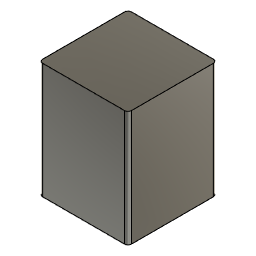
Body v1 (Autodesk Fusion 360 design; units mm, degrees)
Autodesk Fusion 360 part; units mm, degrees
sketch "Sketch1" plane through (0, 0, 0) normal (0, 0, 1) x (1, 0, 0)
  line L0 (25, -25) -> (-25, -25)
  line L1 (-25, -25) -> (-25, 25)
  line L2 (-25, 25) -> (25, 25)
  line L3 (25, 25) -> (25, -25)
  line L4 (25, -25) -> (-25, 25) construction
  line L5 (-25, -25) -> (25, 25) construction
  dimension "d1" = 50
  dimension "d2" = 50
  constraint horizontal L0
  constraint perpendicular L0 L1
  constraint parallel L0 L2
  constraint parallel L1 L3
  constraint coincident L4 origin
  constraint coincident L5 origin
  measures "d1" distance of L1.end L2.end
  measures "d2" distance of L0.end L1.end
extrude "Extrude1" add sketch "Sketch1" along normal blind 65
fillet "Fillet1" radius 2 4 edges at (-25, -25, 32.5) (25, -25, 32.5) (-25, 25, 32.5) (25, 25, 32.5)
shell "Shell1" thickness 1.6 removed faces 1 at (7.6667, -8.3333, 65)
sketch "Sketch2" plane through (0, 0, 65) normal (0, 0, 1) x (-1, 0, 0)
  arc A0 (-23, 23.4) -> (-23.4, 23) centre (-23, 23) ccw
  line L0 (-23, 23.4) -> (23, 23.4)
  arc A1 (23.4, 23) -> (23, 23.4) centre (23, 23) ccw
  line L1 (23.4, 23) -> (23.4, -23)
  arc A2 (23, -23.4) -> (23.4, -23) centre (23, -23) ccw
  line L2 (23, -23.4) -> (-23, -23.4)
  arc A3 (-23.4, -23) -> (-23, -23.4) centre (-23, -23) ccw
  line L3 (-23.4, -23) -> (-23.4, 23)
  arc A4 (-25, -23) -> (-23, -25) centre (-23, -23) ccw
  line L4 (-23, -25) -> (23, -25)
  arc A5 (23, -25) -> (25, -23) centre (23, -23) ccw
  line L5 (25, -23) -> (25, 23)
  arc A6 (25, 23) -> (23, 25) centre (23, 23) ccw
  line L6 (23, 25) -> (-23, 25)
  arc A7 (-23, 25) -> (-25, 23) centre (-23, 23) ccw
  line L7 (-25, 23) -> (-25, -23)
extrude "Extrude2" add sketch "Sketch2" against normal blind 1.6 contours A0 L0 A1 L1 A2 L2 A3 L3
